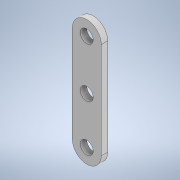
# Autodesk Inventor part: zawieszenie ramie 2
Saved by Autodesk Inventor 2021 (Build 250183000, 183)
## iProperties
Created: 2021-06-25
Part Number: zawieszenie ramie 2
Material: Generic
Document SubType Name: Modeling
Designer: Łukasz
Density: 1 g/cm^3
Appearance: Default
Author: Łukasz
Autodesk Inventor part; units mm, degrees
ref_plane "YZ Plane" through (0, 0, 0) normal (1, 0, 0) x (0, 1, 0)
ref_plane "XZ Plane" through (0, 0, 0) normal (0, 1, 0) x (-1, 0, 0)
ref_plane "XY Plane" through (0, 0, 0) normal (0, 0, 1) x (1, 0, 0)
sketch "Sketch1" plane through (0, 0, 0) normal (0, 0, 1) x (1, 0, 0)
  line L0 (-9, 0) -> (-9, 0)
  line L1 (-18, 9) -> (-18, 69)
  line L2 (-9, 78) -> (-9, 78)
  line L3 (0, 69) -> (0, 9)
  circle A0 centre (-9, 38) radius 4
  arc A1 (-18, 9) -> (-9, 0) centre (-9, 9) ccw
  arc A2 (-9, 0) -> (0, 9) centre (-9, 9) ccw
  arc A3 (0, 69) -> (-9, 78) centre (-9, 69) ccw
  arc A4 (-9, 78) -> (-18, 69) centre (-9, 69) ccw
  circle A5 centre (-9, 9) radius 4
  circle A6 centre (-9, 69) radius 4
  point P0 (0, 0)
  point P1 (-18, 78)
  point P2 (-18, 0)
  point P3 (0, 78)
  dimension "d0" = 18
  dimension "d1" = 78
  dimension "d2" = 8
  dimension "d3" = 9
  dimension "d4" = 8
  dimension "d5" = 8
  constraints: 8 end point, 8 point on circle, 8 point on line, 8 tangent, 7 centre point, 3 equal radius, 2 coincident, 2 parallel, 1 horizontal, 1 perpendicular
  measures "d0" distance of point (-18, 78) point (0, 78)
  measures "d1" distance of point (-18, 0) point (-18, 78)
  measures "d2" diameter of A0
  measures "d3" radius of A1
  measures "d4" diameter of A5
  measures "d5" diameter of A6
extrude "Extrusion1" add sketch "Sketch1" along normal blind 4
body "Solid1"
